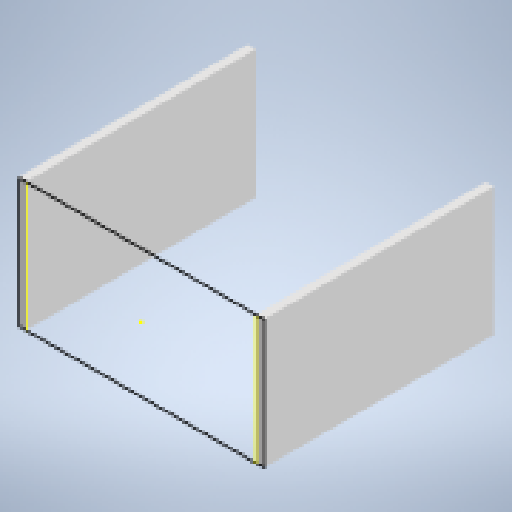
# Autodesk Inventor part: Empujador
Saved by Autodesk Inventor 2024 (Build 280153000, 153)
## iProperties
Created: 2025-03-07
Part Number: Empujador
Material: Genérico
Document SubType Name: Modeling
Designer: sergi
Density: 1 g/cm^3
Appearance: Valor por defecto
Author: sergi
Autodesk Inventor part; units mm, degrees
ref_plane "YZ Plane" through (0, 0, 0) normal (1, 0, 0) x (0, 1, 0)
ref_plane "XZ Plane" through (0, 0, 0) normal (0, 1, 0) x (-1, 0, 0)
ref_plane "XY Plane" through (0, 0, 0) normal (0, 0, 1) x (1, 0, 0)
sketch "Boceto1" plane through (0, 0, 0) normal (0, 0, 1) x (1, 0, 0)
  circle A0 centre (31.4, 31.4) radius 1.6 projected
  circle A1 centre (31.4, -31.4) radius 1.6 projected
  circle A2 centre (-31.4, -31.4) radius 1.6 projected
  circle A3 centre (-31.4, 31.4) radius 1.6 projected
  line L0 (-36.5, 28.5) -> (-36.5, 7) projected
  line L1 (-36.5, 7) -> (-39.5, 7) projected
  line L2 (-39.5, 7) -> (-39.5, -8) projected
  line L3 (-36.5, -8) -> (-39.5, -8) projected
  line L4 (-36.5, -8) -> (-36.5, -28.5) projected
  line L5 (-36.5, -28.5) -> (-44.5, -28.5) projected
  line L6 (-44.5, -26.6905) -> (-44.5, -28.5) projected
  line L7 (-44.5, -26.6905) -> (-47.5, -26.6905) projected
  line L8 (-47.5, -26.6905) -> (-47.5, -38.3095) projected
  line L9 (-44.5, -38.3095) -> (-47.5, -38.3095) projected
  line L10 (-44.5, -36.5) -> (-44.5, -38.3095) projected
  line L11 (44.5, -36.5) -> (-44.5, -36.5) projected
  line L12 (44.5, -36.5) -> (44.5, -38.3095) projected
  line L13 (44.5, -38.3095) -> (47.5, -38.3095) projected
  line L14 (47.5, -26.6905) -> (47.5, -38.3095) projected
  line L15 (44.5, -26.6905) -> (47.5, -26.6905) projected
  line L16 (44.5, -26.6905) -> (44.5, -28.5) projected
  line L17 (36.5, -28.5) -> (44.5, -28.5) projected
  line L18 (36.5, -28.5) -> (36.5, -8) projected
  line L19 (36.5, -8) -> (39.5, -8) projected
  line L20 (39.5, 7) -> (39.5, -8) projected
  line L21 (36.5, 7) -> (39.5, 7) projected
  line L22 (36.5, 7) -> (36.5, 28.5) projected
  line L23 (36.5, 28.5) -> (44.5, 28.5) projected
  line L24 (44.5, 26.6905) -> (44.5, 28.5) projected
  line L25 (44.5, 26.6905) -> (47.5, 26.6905) projected
  line L26 (47.5, 26.6905) -> (47.5, 38.3095) projected
  line L27 (44.5, 38.3095) -> (47.5, 38.3095) projected
  line L28 (44.5, 36.5) -> (44.5, 38.3095) projected
  line L29 (-44.5, 36.5) -> (44.5, 36.5) projected
  line L30 (-44.5, 36.5) -> (-44.5, 38.3095) projected
  line L31 (-44.5, 38.3095) -> (-47.5, 38.3095) projected
  line L32 (-47.5, 26.6905) -> (-47.5, 38.3095) projected
  line L33 (-44.5, 26.6905) -> (-47.5, 26.6905) projected
  line L34 (-44.5, 26.6905) -> (-44.5, 28.5) projected
  line L35 (-36.5, 28.5) -> (-44.5, 28.5) projected
  arc A4 (-24.3254, -32) -> (-32, -24.3254) centre (-31.4, -31.4) ccw projected
  line L36 (-24.3254, -32) -> (24.3254, -32) projected
  arc A5 (32, -24.3254) -> (24.3254, -32) centre (31.4, -31.4) ccw projected
  line L37 (32, -24.3254) -> (32, -21) projected
  line L38 (32, -21) -> (42, -21) projected
  line L39 (42, -23.2697) -> (42, -21) projected
  line L40 (42, -23.2697) -> (45, -23.2697) projected
  line L41 (45, -23.2697) -> (45, -13.7303) projected
  line L42 (42, -13.7303) -> (45, -13.7303) projected
  line L43 (42, -16) -> (42, -13.7303) projected
  line L44 (32, -16) -> (42, -16) projected
  line L45 (32, -16) -> (32, 16) projected
  line L46 (32, 16) -> (42, 16) projected
  line L47 (42, 16) -> (42, 13.7303) projected
  line L48 (42, 13.7303) -> (45, 13.7303) projected
  line L49 (45, 23.2697) -> (45, 13.7303) projected
  line L50 (42, 23.2697) -> (45, 23.2697) projected
  line L51 (42, 23.2697) -> (42, 21) projected
  line L52 (32, 21) -> (42, 21) projected
  line L53 (32, 21) -> (32, 24.3254) projected
  arc A6 (24.3254, 32) -> (32, 24.3254) centre (31.4, 31.4) ccw projected
  line L54 (24.3254, 32) -> (-24.3254, 32) projected
  arc A7 (-32, 24.3254) -> (-24.3254, 32) centre (-31.4, 31.4) ccw projected
  line L55 (-32, 24.3254) -> (-32, 21) projected
  line L56 (-32, 21) -> (-42, 21) projected
  line L57 (-42, 23.2697) -> (-42, 21) projected
  line L58 (-42, 23.2697) -> (-45, 23.2697) projected
  line L59 (-45, 23.2697) -> (-45, 13.7303) projected
  line L60 (-42, 13.7303) -> (-45, 13.7303) projected
  line L61 (-42, 16) -> (-42, 13.7303) projected
  line L62 (-32, 16) -> (-42, 16) projected
  line L63 (-32, 16) -> (-32, -16) projected
  line L64 (-32, -16) -> (-42, -16) projected
  line L65 (-42, -16) -> (-42, -13.7303) projected
  line L66 (-42, -13.7303) -> (-45, -13.7303) projected
  line L67 (-45, -23.2697) -> (-45, -13.7303) projected
  line L68 (-42, -23.2697) -> (-45, -23.2697) projected
  line L69 (-42, -23.2697) -> (-42, -21) projected
  line L70 (-32, -21) -> (-42, -21) projected
  line L71 (-32, -21) -> (-32, -24.3254) projected
  line L72 (-42, -23.5) -> (-45, -23.5)
  line L73 (-45, 23.5) -> (-42, 23.5)
  line L74 (-45, 23.5) -> (-42, 23.5)
  line L75 (-42, 23.5) -> (-42, -23.5)
  line L76 (-42, -23.5) -> (-45, -23.5)
  line L77 (-45, -23.5) -> (-45, 23.5)
  line L78 (42, 23.5) -> (45, 23.5)
  line L79 (45, -23.5) -> (42, -23.5)
  line L80 (42, -23.5) -> (45, -23.5)
  line L81 (45, -23.5) -> (45, 23.5)
  line L82 (45, 23.5) -> (42, 23.5)
  line L83 (42, 23.5) -> (42, -23.5)
  point P0 (0, 0)
  point P1 (-45, -23.5)
  dimension "d0" = 3
  dimension "d1" = 47
  constraints: 24 end point, 4 parallel, 2 horizontal, 2 perpendicular, 12 other
  measures "d0" distance of L75.end L76.end
  measures "d1" distance of L74.end L75.end
ref_plane "Plano de trabajo1" through (-36.5, -36.5, -84) normal (0, 0, -1) x (0.0000001, 1, 0)
extrude "Extrusión1" add sketch "Boceto1" against normal up to surface (84 mm away) contours L75 L61 L60 L59 L58 L57 | L58 L77 L73 L75 | L75 L66 L77 L60 | L65 L75 L69 L68 L67 L66 | L68 L75 L72 L77 | L51 L50 L49 L48 L47 L83 | L83 L78 L81 L50 | L48 L81 L42 L83 | L42 L41 L40 L39 L83 L43 | L81 L79 L83 L40
sketch "Boceto3" plane through (0, 0, 0) normal (0, 0, 1) x (1, 0, 0)
  line L0 (-42, -23.5) -> (-42, 23.5) projected
  line L1 (-42, 23.5) -> (-45, 23.5) projected
  line L2 (-45, 23.5) -> (-45, -23.5) projected
  line L3 (-45, -23.5) -> (-42, -23.5) projected
  line L4 (42, -23.5) -> (45, -23.5) projected
  line L5 (45, -23.5) -> (45, 23.5) projected
  line L6 (45, 23.5) -> (42, 23.5) projected
  line L7 (42, 23.5) -> (42, -23.5) projected
  line L8 (-45, -23.5) -> (45, -23.5)
  line L9 (45, -23.5) -> (45, 23.5)
  line L10 (45, 23.5) -> (-45, 23.5)
  line L11 (-45, 23.5) -> (-45, -23.5)
  point P0 (0, 0)
  constraints: 8 end point, 2 parallel, 1 horizontal, 1 perpendicular
